# Autodesk Inventor part: Roller Chain Sprocket2
Saved by Autodesk Inventor 2016 (Build 200138000, 138)
## iProperties
Created: 2016-04-25
Part Number: Roller Chain Sprocket2
Material: Steel
Document SubType Name: Modeling
Designer: Henrik Samuelsson
Density: 1 g/cm^3
Appearance: Steel
CustomPartVersion: 1
Author: Henrik Samuelsson
Autodesk Inventor part; units mm, degrees
ref_plane "YZ Plane" through (0, 0, 0) normal (1, 0, 0) x (0, 1, 0)
ref_plane "XZ Plane" through (0, 0, 0) normal (0, 1, 0) x (-1, 0, 0)
sketch "Theoretical Tooth Profile" plane through (0, 0, 0) normal (0, 0, 1) x (1, 0, 0)
  circle A0 centre (0, 0) radius 265.1224 construction
  line L0 (0, 0) -> (0, 265.1224) construction
  line L1 (0, 0) -> (29.1656, 263.5133) construction
  circle A1 centre (0, 0) radius 269.6944
  arc A2 (-4.6666, 261.7253) -> (4.6666, 261.7253) centre (0, 265.1224) ccw
  line L2 (0, 265.1224) -> (29.1656, 263.5133) construction
  line L3 (0, 265.1224) -> (7.3927, 270.5039) construction
  line L4 (7.3927, 270.5039) -> (-6.7078, 265.6391) construction
  arc A3 (8.4494, 269.562) -> (7.2628, 267.2477) centre (15.9777, 264.2409) ccw
  arc A4 (-7.2628, 267.2477) -> (-8.4494, 269.562) centre (-15.9777, 264.2409) ccw
  line L5 (-15.9777, 264.2409) -> (-7.2628, 267.2477) construction
  arc A5 (-6.7078, 265.6391) -> (-4.6666, 261.7253) centre (7.3927, 270.5039) ccw
  line L6 (-6.7078, 265.6391) -> (-7.2628, 267.2477)
  arc A6 (4.6666, 261.7253) -> (6.7078, 265.6391) centre (-7.3927, 270.5039) ccw
  line L7 (7.2628, 267.2477) -> (6.7078, 265.6391)
  line L8 (0, 0) -> (14.8569, 269.2849) construction
  point P0 (14.5828, 264.3179)
  dimension "d0" = 530.2448
  dimension "d2" = 6.316
  dimension "d3" = 5.7721
  dimension "d10" = 126.053
  dimension "d11" = 17.017
  dimension "d12" = 9.144
  dimension "d13" = 14.9162
  dimension "d14" = 16.002
  dimension "d23" = 4.9746
  constraints: 18 end point, 15 point on circle, 7 centre point, 3 coincident, 3 point on line, 3 symmetric about line, 3 tangent, 1 equal radius, 1 midpoint, 1 parallel, 1 vertical, 1 other
  measures "d0" diameter of A0
  measures "d2" angle of L1 L0
  measures "d3" radius of A2
  measures "d10" angle of L3 L0
  measures "d11" angle of L4 L3
  measures "d12" distance of L2.start L3.end
  measures "d13" distance of L3.end L4.end
  measures "d14" distance of A3.centre L0.end
  measures "d23" distance from line of L8.end L2
sketch "Tooth Profile" plane through (0, 0, 0) normal (0, 0, 1) x (1, 0, 0)
  circle A0 centre (0, 0) radius 269.6944 projected
  line L0 (0, 0) -> (0, 265.1224) construction
  line L1 (0, 265.1224) -> (5.3963, 263.0737) construction
  arc A1 (-5.3963, 263.0737) -> (5.3963, 263.0737) centre (0, 265.1224) ccw
  line L2 (-5.3963, 263.0737) -> (0, 265.1224) construction
  arc A2 (-5.3963, 263.0737) -> (-8.1933, 269.5699) centre (-81.0518, 234.3508) ccw
  arc A3 (8.1933, 269.5699) -> (5.3963, 263.0737) centre (81.0518, 234.3508) ccw
  dimension "d44" = 138.421
  dimension "d45" = 5.7721
  dimension "d46" = 80.9244
  constraints: 8 point on circle, 7 end point, 3 centre point, 2 tangent, 1 coincident, 1 equal radius, 1 symmetric about line, 1 vertical
  measures "d44" angle of L1 L2
  measures "d45" radius of A1
  measures "d46" radius of A3
sketch "Section Profile" plane through (0, 0, 0) normal (1, 0, 0) x (0, 1, 0)
  line L0 (269.6944, 0) -> (-269.6944, 0) projected
  line L1 (252.6298, 7.4636) -> (-252.6298, 7.4636)
  line L2 (-252.6298, 7.4636) -> (-252.6298, -7.4636)
  line L3 (-252.6298, -7.4636) -> (252.6298, -7.4636)
  line L4 (252.6298, -7.4636) -> (252.6298, 7.4636)
  line L5 (252.6298, 7.4636) -> (269.6944, 7.4636) construction
  line L6 (269.6944, 7.4636) -> (269.6944, -7.4636) construction
  line L7 (269.6944, -7.4636) -> (252.6298, -7.4636) construction
  line L8 (252.6298, -7.4636) -> (252.6298, 7.4636)
  arc A0 (269.6944, 4.6274) -> (259.7117, 7.4636) centre (259.7117, -11.5229) ccw
  arc A1 (259.7117, -7.4636) -> (269.6944, -4.6274) centre (259.7117, 11.5229) ccw
  line L9 (259.7117, 7.4636) -> (0, 7.4636)
  line L10 (0, 7.4636) -> (0, -7.4636)
  line L11 (0, -7.4636) -> (259.7117, -7.4636)
  line L12 (0, 7.4636) -> (0, -7.4636)
  line L13 (269.6944, 4.6274) -> (269.6944, -4.6274)
  point P0 (0, 0)
  point P1 (0, 0)
  dimension "d30" = 14.9272
  dimension "d31" = 505.2597
  dimension "d32" = 14.9272
  dimension "d33" = 2.8362
  dimension "d34" = 18.9865
  dimension "d43" = 7.4636
  constraints: 26 end point, 7 midpoint, 5 perpendicular, 4 parallel, 4 point on circle, 3 point on line, 3 symmetric about line, 2 centre point, 2 horizontal, 2 tangent, 1 collinear, 1 other
  measures "d30" distance between parallel lines of L7 L5
  measures "d31" distance between parallel lines of L2 L4
  measures "d32" distance between parallel lines of L3 L1
  measures "d33" distance from line of L13.start L5
  measures "d34" radius of A0
  measures "d43" distance between parallel lines of L3 L0
revolve "Shroud" add sketch "Section Profile" angle 360 about axis through (0, 0, 7.4636) along (0, 0, -1) contours L10 L3 L2 L0 | L0 L2 L1 L10
revolve "Strand" add sketch "Section Profile" angle 360 about axis through (0, 0, 7.4636) along (0, 0, -1) contours L13 A1 L11 L4 L0 | L0 L4 L9 A0 L13 | L4 L3 L10 L0 | L0 L10 L1 L4
pattern_of_one "Strand Pattern"
extrude "Theoretical Tooth" cut sketch "Theoretical Tooth Profile" along normal through all both and the other way through all contours A3 L7 A6 A2 A5 L6 A4 A1 picked at (0, 266.2366)
extrude "Tooth" [suppressed]
pattern_circular "Tooth Pattern" count 57 over 360 about axis through (0, 0, -10) along (0, 0, 1) of "Theoretical Tooth"
ref_plane "Timing Plane" through (0, 265.1224, 0) normal (1, 0, 0) x (0, 1, 0)
equation "\"d3\" = 0.5 * da_Dr + da_SC"
equation "\"d12\" = 0.8 * da_Dr"
equation "\"d13\" = 1.3 * da_Dr + da_SC"
equation "\"d14\" = 1.4 * da_Dr"
equation "\"d23\" = da_Ha"
equation "\"d44\" = da_Alfa"
equation "\"d45\" = da_Ri"
equation "\"d46\" = da_Re"
equation "\"d30\" = da_Bf"
equation "\"d31\" = da_Ds"
equation "\"d32\" = da_Bs"
equation "\"d33\" = da_Ba"
equation "\"d34\" = da_Rx"
equation "\"d40\" = da_pt"
equation "\"form_type\" = 0"
equation "\"da_p\" = 29.21"
equation "\"da_Dr\" = 11.43"
equation "\"da_SC\" = 0.05715"
equation "\"da_Ha\" = 4.97458"
equation "\"da_pt\" = 25"
equation "\"da_Bf\" = 14.9272"
equation "\"da_Ba\" = 2.83617"
equation "\"da_Rx\" = 18.9865"
equation "\"da_Ra\" = 1.27"
equation "\"da_Bs\" = 14.9272"
equation "\"da_Ds\" = 505.25966"
equation "\"da_Re\" = 80.9244"
equation "\"da_Ri\" = 5.77215"
equation "\"da_Alfa\" = 138.421deg"
body "Solid1"
